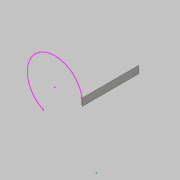
# Autodesk Inventor part: duck
Saved by Autodesk Inventor 2016 (Build 200138000, 138)
## iProperties
Created: 2016-03-14
Part Number: duck
Material: Generic
Document SubType Name: Modeling
Designer: Ritz
Density: 1 g/cm^3
Appearance: Default
Author: Ritz
Autodesk Inventor part; units mm, degrees
ref_plane "YZ Plane" through (0, 0, 0) normal (1, 0, 0) x (0, 1, 0)
ref_plane "XZ Plane" through (0, 0, 0) normal (0, 1, 0) x (-1, 0, 0)
ref_plane "XY Plane" through (0, 0, 0) normal (0, 0, 1) x (1, 0, 0)
sketch "Sketch1" plane through (0, 0, 0) normal (0, 0, 1) x (1, 0, 0)
  arc A0 (-3.8854, 15.6814) -> (16.1434, 0.6264) centre (11.2356, 14.9476) ccw
  arc A1 (-3.8854, 15.6814) -> (-3.915, 15.674) centre (0, 0) ccw
  arc A2 (-14.2514, 7.6093) -> (16.1434, 0.6264) centre (0, 0) ccw
  arc A3 (-3.915, 15.674) -> (-18.3827, 16.4116) centre (-11.2328, 14.3967) ccw
  arc A4 (-3.8449, 13.6212) -> (-3.8918, 15.5333) centre (-11.2328, 14.3967) ccw
  line L0 (-18.3827, 16.4116) -> (-14.2514, 7.6093)
  circle A5 centre (-12.1999, 18.1336) radius 1.555
  ellipse E0 centre (-1.0981, -5.3272) end of major axis (8.9522, -10.3074) minor radius 1.7466
  constraints: 12 point on circle, 6 centre point, 2 coincident, 2 end point, 2 other
extrude "Extrusion1" add sketch "Sketch1" along normal blind 15.24 contours A4 A0
sketch "Sketch3" plane through (0, 0, 15.24) normal (0, 0, 1) x (1, 0, 0)
  arc A0 (-3.915, 15.674) -> (-14.2514, 7.6093) centre (-11.2328, 14.3967) ccw projected
  point P0 (0, 0)
body "Solid1"
